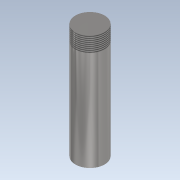
# Autodesk Inventor part: pasador
Saved by Autodesk Inventor 2021 (Build 250183000, 183)
## iProperties
Created: 2021-06-18
Part Number: pasador
Material: Steel, Carbon
Document SubType Name: Modeling
Designer: Andrés Holguín
Density: 7.85 g/cm^3
Appearance: Semi-Polished
Author: Andrés Holguín
Autodesk Inventor part; units mm, degrees
ref_plane "YZ Plane" through (0, 0, 0) normal (1, 0, 0) x (0, 1, 0)
ref_plane "XZ Plane" through (0, 0, 0) normal (0, 1, 0) x (-1, 0, 0)
ref_plane "XY Plane" through (0, 0, 0) normal (0, 0, 1) x (1, 0, 0)
sketch "Sketch1" plane through (0, 0, 0) normal (0, 1, 0) x (-1, 0, 0)
  circle A0 centre (0, 0) radius 12.7
  dimension "d0" = 25.4
  constraints: 1 centre point, 1 coincident
  measures "d0" diameter of A0
extrude "Extrusion1" add sketch "Sketch1" along normal blind 105
thread "Thread1" size "M26x1.5" class "6g" standard "ANSI Metric M Profile" length 15
body "Solid1"
